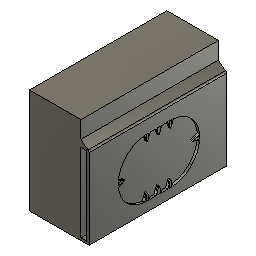
2nd mirror calibration holder with tabs (Autodesk Fusion 360 design; units mm, degrees)
Autodesk Fusion 360 part; units mm, degrees
sketch "Sketch1" plane through (0, 0, 0) normal (1, 0, 0) x (0, 0, -1)
  line L0 (0, 0) -> (-57, 0)
  line L1 (-57, 0) -> (-57, 54)
  line L2 (-57, 54) -> (0, 54)
  line L3 (0, 54) -> (0, 0)
  dimension "d1" = 57
  dimension "d2" = 54
  constraint horizontal L0
  constraint vertical L1
  constraint horizontal L2
  constraint vertical L3
  constraint coincident L0.start L3.end
  measures "d1" distance of L0.start L0.end
  measures "d2" distance of L0.start L2.end
extrude "Extrude1" add sketch "Sketch1" along normal blind 9 makes body 1
sketch "Sketch2" plane through (9, 0, 0) normal (1, 0, 0) x (0, 0, -1)
  line L0 (0, 54) -> (-57, 54)
  line L1 (-57, 54) -> (-57, 0)
  line L2 (-57, 0) -> (0, 0)
  line L3 (0, 0) -> (0, 54)
  circle A0 centre (-28, 27) radius 18.5
  circle A1 centre (-28, 27) radius 12.5 construction
  line L4 (-28, 27) -> (-23, 27) construction
  line L5 (-28, 27) -> (-33, 27) construction
  circle A2 centre (-23, 27) radius 12.5
  circle A3 centre (-33, 27) radius 12.5
  line L6 (-45.5, 27) -> (-42.5, 27)
  line L7 (-42.5, 27) -> (-45.4405, 28.218)
  line L8 (-42.5, 27) -> (-45.4405, 25.782)
  line L9 (-33, 17.5) -> (-31.782, 14.5595)
  line L10 (-33, 14.5) -> (-33, 17.5) construction
  line L11 (-33, 17.5) -> (-34.218, 14.5595)
  line L12 (-33, 39.5) -> (-33, 36.5) construction
  line L13 (-33, 36.5) -> (-34.218, 39.4405)
  line L14 (-33, 36.5) -> (-31.782, 39.4405)
  line L15 (-28, 36.5) -> (-29.218, 39.4405)
  line L16 (-28, 39.5) -> (-28, 36.5) construction
  line L17 (-28, 36.5) -> (-26.782, 39.4405)
  line L18 (-28, 17.5) -> (-29.218, 14.5595)
  line L19 (-28, 14.5) -> (-28, 17.5) construction
  line L20 (-28, 17.5) -> (-26.782, 14.5595)
  line L21 (-23, 36.5) -> (-24.218, 39.4405)
  line L22 (-23, 39.5) -> (-23, 36.5) construction
  line L23 (-23, 36.5) -> (-21.782, 39.4405)
  line L24 (-23, 17.5) -> (-24.218, 14.5595)
  line L25 (-23, 14.5) -> (-23, 17.5) construction
  line L26 (-23, 17.5) -> (-21.782, 14.5595)
  line L27 (-45.5, 27) -> (-42.5, 27) construction
  line L28 (-42.5, 27) -> (-45.4405, 28.218)
  line L29 (-42.5, 27) -> (-45.4405, 25.782)
  line L30 (-10.5, 27) -> (-13.5, 27) construction
  line L31 (-13.5, 27) -> (-10.5595, 25.782)
  line L32 (-13.5, 27) -> (-10.5595, 28.218)
  line L33 (-33, 39.5) -> (-23, 39.5)
  line L34 (-33, 14.5) -> (-23, 14.5)
  line L35 (-31.782, 14.5595) -> (-31.7574, 14.5)
  line L36 (-29.218, 14.5595) -> (-29.2426, 14.5)
  line L37 (-26.782, 14.5595) -> (-26.7574, 14.5)
  line L38 (-24.218, 14.5595) -> (-24.2426, 14.5)
  line L39 (-31.782, 39.4405) -> (-31.7574, 39.5)
  line L40 (-29.218, 39.4405) -> (-29.2426, 39.5)
  line L41 (-26.782, 39.4405) -> (-26.7574, 39.5)
  line L42 (-24.218, 39.4405) -> (-24.2426, 39.5)
  dimension "d5" = 37
  dimension "d6" = 25
  dimension "d127" = 5
  dimension "d128" = 5
  dimension "d129" = 25
  dimension "d130" = 25
  dimension "d131" = 45
  dimension "d132" = 3
  dimension "d133" = 45
  dimension "d134" = 3
  dimension "d135" = 45
  dimension "d136" = 3
  dimension "d140" = 45
  dimension "d141" = 3
  dimension "d142" = 45
  dimension "d143" = 3
  dimension "d144" = 45
  dimension "d145" = 3
  dimension "d146" = 45
  dimension "d147" = 3
  dimension "d148" = 45
  dimension "d149" = 3
  dimension "d150" = 3
  dimension "d151" = 45
  constraint concentric A0 A1
  constraint coincident A0.centre A1.centre
  constraint horizontal L4
  constraint parallel L4 L5
  constraint coincident L4.end A2.centre
  constraint coincident L5.end A3.centre
  constraint coincident A3 L6.start
  constraint horizontal L6
  constraint coincident A3 L7.end
  constraint collinear L5 L6
  constraint symmetric L7.start L6 L8.start
  constraint symmetric L9.start L11.start L10
  constraint symmetric L9.end L11.end L10
  constraint symmetric L13.start L14.start L12
  constraint symmetric L13.end L14.end L12
  constraint coincident A3 L12.start
  constraint coincident A3 L13.end
  constraint vertical L12
  constraint coincident A3 L14.end
  constraint coincident A3 L11.end
  constraint coincident A3 L10.start
  constraint coincident A3 L9.end
  constraint vertical L10
  constraint coincident A3 L8.end
  constraint equal L7 L8
  constraint symmetric L18.start L20.start L19
  constraint symmetric L18.end L20.end L19
  constraint symmetric L15.start L17.start L16
  constraint symmetric L15.end L17.end L16
  constraint vertical L16
  constraint vertical L19
  constraint symmetric L24.start L26.start L25
  constraint symmetric L24.end L26.end L25
  constraint symmetric L21.start L23.start L22
  constraint symmetric L21.end L23.end L22
  constraint vertical L22
  constraint vertical L25
  constraint horizontal L27
  constraint symmetric L6.end L7.start L27
  constraint equal L28 L29
  constraint coincident A1 L15.end
  constraint coincident A1 L16.start
  constraint coincident A1 L17.end
  constraint coincident A2 L21.end
  constraint coincident A2 L22.start
  constraint coincident A2 L23.end
  constraint coincident A2 L32.end
  constraint coincident A2 L30.start
  constraint coincident A2 L31.end
  constraint horizontal L30
  constraint symmetric L30 L31 L32
  constraint coincident L30.end L32
  constraint coincident L31.start L30
  constraint equal L31 L32
  constraint coincident A1 L18.end
  constraint coincident A1 L19.start
  constraint coincident A1 L20.end
  constraint coincident A2 L24.end
  constraint coincident A2 L25.start
  constraint coincident A2 L26.end
  constraint coincident L34 L35.end
  constraint parallel L9 L35
  constraint coincident L34 L36.end
  constraint parallel L18 L36
  constraint coincident L34 L37.end
  constraint parallel L20 L37
  constraint coincident L34 L38.end
  constraint parallel L24 L38
  constraint coincident L33 L39.end
  constraint parallel L14 L39
  constraint coincident L33 L40.end
  constraint parallel L15 L40
  constraint coincident L33 L41.end
  constraint parallel L17 L41
  constraint coincident L33 L42.end
  constraint parallel L21 L42
  measures "d5" diameter of A0
  measures "d6" diameter of A1
  measures "d127" distance of A0.centre L5.end
  measures "d128" distance of A0.centre L4.end
  measures "d129" diameter of A2
  measures "d130" diameter of A3
  measures "d131" angle of L7 L8
  measures "d132" distance of L6.start L6.end
  measures "d133" angle of L9 L11
  measures "d134" distance of L9.start L10.start
  measures "d135" angle of L13 L14
  measures "d136" distance of L12.end L12.start
  measures "d140" angle of L18 L20
  measures "d141" distance of L18.start L19.start
  measures "d142" angle of L15 L17
  measures "d143" distance of L16.start L15.start
  measures "d144" angle of L24 L26
  measures "d145" distance of L24.start L25.start
  measures "d146" angle of L21 L23
  measures "d147" distance of L21.start L22.start
  measures "d148" angle of L28 L29
  measures "d149" distance of L6.end L6.start
  measures "d150" distance of L30.end L30.start
  measures "d151" angle of L31 L32
extrude "Extrude16" cut sketch "Sketch2" against normal blind 1 contours A2 A3 L17 L20 L21 L23 L24 L26 L31 L32 | A2 L17 L33 L41 L42 | A2 L20 L34 L37 L38 | A2 A3 L15 L17 L18 L20 | A3 L15 L33 L39 L40 | A3 L18 L34 L35 L36 | A2 A3 L7 L8 L9 L11 L13 L14 L15 L18 L28 L29 bodies 1
sketch "Sketch3" plane through (9, 27, 28) normal (1, 0, 0) x (0, 0, -1)
  line L0 (-29.01, 27.5) -> (28.01, 27.5)
  line L1 (28.01, 27.5) -> (28.01, -26.5)
  line L2 (-29.01, 27.5) -> (-29.01, -26.5)
  line L3 (28, 27) -> (-29, 27)
  line L4 (-29, 27) -> (-29, -27)
  line L5 (28, -27) -> (28, 27)
  line L6 (-30.01, 28.5) -> (-30.01, -26.5)
  line L7 (-30.01, 28.5) -> (29.01, 28.5)
  line L8 (29.01, 28.5) -> (29.01, -26.5)
  line L9 (-30.01, -26.5) -> (-29.01, -26.5)
  line L10 (29.01, -26.5) -> (28.01, -26.5)
  dimension "d7" = 0.5
  dimension "d8" = 0.01
  dimension "d9" = 0.01
  dimension "d10" = 54
  dimension "d11" = -1
  constraint horizontal L0
  constraint perpendicular L0 L1
  constraint perpendicular L0 L2
  constraint equal L1 L2
  constraint perpendicular L2 L9
  constraint perpendicular L1 L10
  measures "d7" distance of L0 L3
  measures "d8" distance of L2 L4
  measures "d9" distance of L1 L5
  measures "d10" distance of L0.start L2.end
extrude "Extrude2" add sketch "Sketch3" along normal blind -9.8 and the other way blind -0.8 separate body makes body 2
sketch "Sketch4" plane through (0, 0, -0.01) normal (0, 0, 1) x (1, 0, 0)
  line L0 (9.8, 54.5) -> (-0.8, 54.5)
  line L1 (-0.8, 54.5) -> (-0.8, 0.5)
  line L2 (-0.8, 0.5) -> (9.8, 0.5)
  line L3 (9.8, 0.5) -> (9.8, 54.5)
  line L4 (0, 54.5) -> (0, 0.5)
  line L5 (9, 0.5) -> (9, 54.5)
extrude "Extrude3" add sketch "Sketch4" along normal blind 2 contours L0 L2 L3 L5 | L0 L1 L2 L4 bodies 2
sketch "Sketch5" plane through (0, 54.5, 0) normal (0, -1, 0) x (1, 0, 0)
  line L0 (9, 1.99) -> (9.8, 1.99)
  line L1 (0, 1.99) -> (0, -0.01)
  line L2 (0, -0.01) -> (9, -0.01)
  line L3 (9.8, 1.99) -> (9.8, 57.01)
  line L4 (9.8, 57.01) -> (-0.8, 57.01)
  line L5 (-0.8, 57.01) -> (-0.8, 1.99)
  line L6 (0, 57.01) -> (0, 1.99)
  line L7 (9, -0.01) -> (9, 1.99)
  line L8 (9, 1.99) -> (9, 57.01)
  line L9 (-0.8, 1.99) -> (0, 1.99)
extrude "Extrude4" add sketch "Sketch5" along normal blind 2 contours L4 L5 L6 L9 bodies 2
sketch "Sketch6" plane through (0, 0, 57.01) normal (0, 0, -1) x (-1, 0, 0)
  line L0 (0.8, 52.5) -> (0, 52.5)
  line L1 (0, 52.5) -> (0, 54.5)
  line L2 (0, 54.5) -> (-9.8, 54.5)
  line L3 (-9.8, 54.5) -> (-9.8, 0.5)
  line L4 (-9.8, 0.5) -> (0.8, 0.5)
  line L5 (0.8, 0.5) -> (0.8, 52.5)
  line L6 (0, 0.5) -> (0, 52.5)
  line L7 (-9, 54.5) -> (-9, 0.5)
extrude "Extrude5" add sketch "Sketch6" along normal blind 2 contours L0 L4 L5 L6 | L2 L3 L4 L7 bodies 2
sketch "Sketch16" plane through (0, 55.5, 0) normal (0, 1, 0) x (-1, 0, 0)
  line L0 (-9.8, -1.01) -> (0.8, -1.01)
  line L1 (0.8, -1.01) -> (0.8, 58.01)
  line L2 (0.8, 58.01) -> (-9.8, 58.01)
  line L3 (-9.8, 58.01) -> (-9.8, -1.01)
  line L4 (-9.8, 58.01) -> (-24.8, 58.01)
  line L5 (-24.8, 58.01) -> (-24.8, -1.01)
  line L6 (-24.8, -1.01) -> (-9.8, -1.01)
  line L7 (-9.8, -1.01) -> (-9.8, 58.01)
  dimension "d81" = 15
  constraint horizontal L4
  constraint vertical L5
  constraint horizontal L6
  constraint vertical L7
  constraint coincident L2.end L3.start
  constraint coincident L0.start L3.end
  measures "d81" distance of L2.end L4.end
extrude "Extrude18" add sketch "Sketch16" against normal blind 1 contours L3 L4 L5 L6 L7 bodies 2
sketch "Sketch17" plane through (0, 54.5, 0) normal (0, -1, 0) x (1, 0, 0)
  line L0 (9.8, 55.01) -> (9, 55.01)
  line L1 (9, 55.01) -> (9, 57.01)
  line L2 (9, 57.01) -> (0, 57.01)
  line L3 (0, 57.01) -> (0, -0.01)
  line L4 (0, -0.01) -> (9, -0.01)
  line L5 (9, -0.01) -> (9, 1.99)
  line L6 (9, 1.99) -> (9.8, 1.99)
  line L7 (9.8, 1.99) -> (9.8, -1.01)
  line L8 (9.8, -1.01) -> (24.8, -1.01)
  line L9 (24.8, -1.01) -> (24.8, 58.01)
  line L10 (24.8, 58.01) -> (9.8, 58.01)
  line L11 (9.8, 58.01) -> (9.8, 55.01)
  line L12 (24.8, -1.01) -> (9.8, -1.01)
  line L13 (9.8, -1.01) -> (9.8, -0.01)
  line L14 (9.8, -0.01) -> (24.8, -0.01)
  line L15 (24.8, -0.01) -> (24.8, -1.01)
  line L16 (24.8, 58.01) -> (9.8, 58.01)
  line L17 (9.8, 58.01) -> (9.8, 57.01)
  line L18 (9.8, 57.01) -> (24.8, 57.01)
  line L19 (24.8, 57.01) -> (24.8, 58.01)
  dimension "d84" = 1
  dimension "d85" = 1
  constraint horizontal L12
  constraint vertical L13
  constraint horizontal L14
  constraint vertical L15
  constraint coincident L7 L13.end
  constraint coincident L8.end L9.start
  constraint horizontal L16
  constraint vertical L17
  constraint horizontal L18
  constraint vertical L19
  constraint coincident L11 L17.end
  constraint coincident L9.end L10.start
  measures "d84" distance of L12 L14
  measures "d85" distance of L9.end L18.end
extrude "Extrude19" add sketch "Sketch17" along normal up to surface (54 mm away) contours L9 L10 L11 L16 L17 L18 L19 | L7 L8 L9 L12 L13 L14 L15 bodies 2
sketch "Sketch19" plane through (0, 54.5, 0) normal (0, -1, 0) x (1, 0, 0)
  line L0 (24.8, -0.01) -> (23.8, -0.01)
  line L1 (23.8, -0.01) -> (23.8, 57.01)
  line L2 (23.8, 57.01) -> (24.8, 57.01)
  line L3 (24.8, 57.01) -> (24.8, -0.01)
  line L4 (21.3, 57.7) -> (19.3, 57.7)
  line L5 (19.3, 57.7) -> (19.3, -0.01)
  line L6 (19.3, -0.01) -> (21.3, -0.01)
  line L7 (21.3, -0.01) -> (21.3, 57.7)
  line L8 (24.8, 57.01) -> (9.8, 57.01)
  line L9 (9.8, 57.01) -> (9.8, 55.01)
  line L10 (9.8, 55.01) -> (9, 55.01)
  line L11 (9, 55.01) -> (9, 57.01)
  line L12 (9, 57.01) -> (0, 57.01)
  line L13 (0, 57.01) -> (0, -0.01)
  line L14 (0, -0.01) -> (9, -0.01)
  line L15 (9, -0.01) -> (9, 1.99)
  line L16 (9, 1.99) -> (9.8, 1.99)
  line L17 (9.8, 1.99) -> (9.8, -0.01)
  line L18 (9.8, -0.01) -> (24.8, -0.01)
  line L19 (24.8, -0.01) -> (24.8, 57.01)
  dimension "d89" = 1
  dimension "d90" = 2
  dimension "d91" = 2.5
  constraint horizontal L0
  constraint vertical L1
  constraint horizontal L2
  constraint vertical L3
  constraint horizontal L4
  constraint vertical L5
  constraint horizontal L6
  constraint vertical L7
  constraint collinear L2 L8
  constraint collinear L0 L18
  constraint collinear L6 L18
  constraint collinear L3 L19
  measures "d89" distance of L1 L3
  measures "d90" distance of L5 L7
  measures "d91" distance of L1 L7
extrude "Extrude20" add sketch "Sketch19" along normal blind 60 contours L0 L1 L2 L3 L8 L18 L19 | L5 L6 L7 L8 L18 bodies 2
extrude "Extrude21" cut 1 faces at (8, 27, 19.8333) along direction (1, 0, 0) up to surface (1 mm away) from surface at 15.8 on bodies 1 bodies 2
sketch "Sketch25" plane through (0, 0, -0.01) normal (0, 0, 1) x (1, 0, 0)
  line L0 (21.3, 0.5) -> (23.8, 0.5)
  line L1 (23.8, 54.5) -> (21.3, 54.5)
  line L2 (24.8, 55.5) -> (24.8, 45.5)
  line L3 (24.8, 45.5) -> (21.3, 45.5)
  line L4 (21.3, 54.5) -> (21.3, 45.5)
  line L5 (24.8, 45.5) -> (24.8, 55.5)
  line L6 (24.8, 55.5) -> (24.8, 0.5)
  line L7 (-0.8, 55.5) -> (24.8, 55.5)
  line L8 (21.3, 54.5) -> (21.3, 55.5)
  line L9 (24.8, 55.5) -> (21.3, 55.5)
  line L10 (24.8, 10.5) -> (19.3, 10.5)
  line L11 (19.3, -5.5) -> (24.8, -5.5)
  line L12 (24.8, -5.5) -> (24.8, 10.5)
  line L13 (9.8, 0.5) -> (19.3, -5.5)
  line L14 (19.3, 0.5) -> (19.3, 54.5)
  line L15 (-0.8, 0.5) -> (24.8, 0.5)
  line L16 (9.8, 0.5) -> (9.8, 54.5)
  line L17 (19.3, 10.5) -> (9.8, 10.5)
  line L18 (9.8, 10.5) -> (9.8, 0.5)
  line L19 (9.8, 0.5) -> (19.3, 0.5)
  line L20 (19.3, 0.5) -> (19.3, 10.5)
  line L21 (9.8, 0.5) -> (9.8, 10.5)
  line L22 (23.8, 0.5) -> (23.8, 54.5)
  line L23 (21.3, 54.5) -> (21.3, 0.5)
  point P0 (19.3, -5.5)
  dimension "d119" = 10
  dimension "d120" = 10
  constraint coincident L1.end L4.start
  constraint coincident L2.end L6
  constraint coincident L2.start L7
  constraint coincident L7 L8.end
  constraint perpendicular L7 L8
  constraint perpendicular L5 L9
  constraint horizontal L3
  constraint horizontal L10
  constraint horizontal L11
  constraint vertical L12
  constraint coincident L6 L10.start
  constraint coincident P0 L11.start
  constraint coincident L10.end L14
  constraint coincident L13.start L15
  constraint coincident L13.start L16
  constraint horizontal L17
  constraint vertical L18
  constraint horizontal L19
  constraint vertical L20
  constraint coincident L13.start L16.start
  measures "d119" distance of L3 L7
  measures "d120" distance of L10 L15
extrude "Extrude26" cut sketch "Sketch25" along normal blind 65 and the other way blind 10 contours L0 L10 L15 L22 L23 | L0 L11 L12 L13 L15 L19 | L10 L14 L15 L20 L23 | L6 L10 L12 L15 L22 | L14 L15 L16 L17 L18 L19 L20 L21 | L1 L3 L4 L22 L23 | L1 L2 L3 L5 L6 L7 L8 L9 L22 bodies 2
sketch "Sketch26" plane through (0, 0, 58.01) normal (0, 0, 1) x (1, 0, 0)
  line L0 (21.3, 55.5) -> (-0.8, 55.5)
  line L1 (-0.8, 55.5) -> (-0.8, 0.5)
  line L2 (-0.8, 0.5) -> (9.8, 0.5)
  line L3 (24.8, 45.5) -> (21.3, 45.5)
  arc A0 (21.3, 48.178) -> (24.8, 45.5) centre (41.2309, 70.6003) ccw
  line L4 (24.8, 10.5) -> (19.3, 10.5)
  line L5 (19.3, 11.5) -> (24.8, 11.5)
  line L6 (24.8, 11.5) -> (24.8, 10.5)
  line L7 (9.8, 0.5) -> (9.8, 10.5)
  line L8 (19.3, 10.5) -> (19.3, 11.5)
  line L9 (24.8, 45.5) -> (21.3, 45.5)
  line L10 (21.3, 45.5) -> (21.3, 55.5)
  line L11 (9.8, 10.5) -> (24.8, 10.5)
  line L12 (24.8, 10.5) -> (24.8, 45.5)
  dimension "d116" = 30
  dimension "d124" = 5.5
  dimension "d125" = 1
  constraint perpendicular L4 L6
  constraint perpendicular L5 L8
  measures "d116" radius of A0
  measures "d124" distance of L6 L8
  measures "d125" distance of L4 L5
extrude "Extrude27" add sketch "Sketch26" against normal up to surface (59.02 mm away) contours L3 A0 L9 L10 | L4 L5 L6 L8 L11 L12 bodies 2
sketch "Sketch27" plane through (0, 0, 58.01) normal (0, 0, 1) x (1, 0, 0)
  line L0 (21.3, 48.178) -> (21.3, 55.5)
  line L1 (24.8, 10.5) -> (24.8, 45.5)
  line L2 (23.7987, 11.5) -> (21.2974, 11.5)
  line L3 (21.2974, 11.5) -> (21.2974, 45.1898)
  line L4 (21.2974, 45.1898) -> (23.7987, 45.1898)
  line L5 (23.7987, 45.1898) -> (23.7987, 11.5)
  line L6 (9.8, 10.5) -> (24.8, 10.5)
  line L7 (9.8, 10.5) -> (-0.8, 10.5)
  line L8 (-0.8, 10.5) -> (-0.8, 0.5)
  line L9 (-0.8, 0.5) -> (9.8, 0.5)
  line L10 (9.8, 0.5) -> (9.8, 10.5)
  arc A0 (21.3, 48.178) -> (24.8, 45.5) centre (41.2309, 70.6003) ccw
  line L11 (21.3, 55.5) -> (-0.8, 55.5)
  line L12 (-0.8, 55.5) -> (-0.8, 0.5)
  line L13 (-0.8, 0.5) -> (9.8, 0.5)
  line L14 (9.8, 0.5) -> (9.8, 10.5)
  dimension "d126" = 1
  constraint horizontal L2
  constraint vertical L3
  constraint horizontal L4
  constraint vertical L5
  constraint horizontal L7
  constraint vertical L8
  constraint horizontal L9
  constraint vertical L10
  constraint coincident L6.start L7.start
  measures "d126" distance of L2 L6
extrude "Extrude28" cut sketch "Sketch27" against normal blind 70 contours L7 L8 L9 L10 L12 L13 L14 | L2 L3 L4 L5 bodies 2
fillet "Fillet3" radius 1 1 edges at (24.8, 45.5, 28.5) on bodies 2
sketch "Sketch28" plane through (24.8, 0, 0) normal (1, 0, 0) x (0, 0, -1)
  line L0 (1.01, 44.9651) -> (-58.01, 44.9651)
  line L1 (-58.01, 44.9651) -> (-58.01, 10.5)
  line L2 (-58.01, 10.5) -> (1.01, 10.5)
  line L3 (1.01, 10.5) -> (1.01, 44.9651)
  arc A0 (-45.4405, 25.782) -> (-34.218, 14.5595) centre (-33, 27) ccw
  line L4 (-45.4405, 25.782) -> (-42.5, 27)
  line L5 (-42.5, 27) -> (-45.4405, 28.218)
  arc A1 (-34.218, 39.4405) -> (-45.4405, 28.218) centre (-33, 27) ccw
  line L6 (-34.218, 39.4405) -> (-33, 36.5)
  line L7 (-33, 36.5) -> (-31.7574, 39.5)
  line L8 (-31.7574, 39.5) -> (-29.2426, 39.5)
  line L9 (-29.2426, 39.5) -> (-28, 36.5)
  line L10 (-28, 36.5) -> (-26.7574, 39.5)
  line L11 (-26.7574, 39.5) -> (-24.2426, 39.5)
  line L12 (-24.2426, 39.5) -> (-23, 36.5)
  line L13 (-23, 36.5) -> (-21.782, 39.4405)
  arc A2 (-10.5595, 28.218) -> (-21.782, 39.4405) centre (-23, 27) ccw
  line L14 (-10.5595, 28.218) -> (-13.5, 27)
  line L15 (-13.5, 27) -> (-10.5595, 25.782)
  arc A3 (-21.782, 14.5595) -> (-10.5595, 25.782) centre (-23, 27) ccw
  line L16 (-21.782, 14.5595) -> (-23, 17.5)
  line L17 (-23, 17.5) -> (-24.2426, 14.5)
  line L18 (-24.2426, 14.5) -> (-26.7574, 14.5)
  line L19 (-26.7574, 14.5) -> (-28, 17.5)
  line L20 (-28, 17.5) -> (-29.2426, 14.5)
  line L21 (-29.2426, 14.5) -> (-31.7574, 14.5)
  line L22 (-31.7574, 14.5) -> (-33, 17.5)
  line L23 (-33, 17.5) -> (-34.218, 14.5595)
  line L24 (-45.4405, 39.5) -> (-10.5595, 39.5)
  line L25 (-10.5595, 39.5) -> (-10.5595, 14.5)
  line L26 (-10.5595, 14.5) -> (-45.4405, 14.5)
  line L27 (-45.4405, 14.5) -> (-45.4405, 39.5)
  line L28 (-42.5, 27.5) -> (-45.4405, 27.5)
  line L29 (-45.4405, 27.5) -> (-45.4405, 26.5)
  line L30 (-45.4405, 26.5) -> (-42.5, 26.5)
  line L31 (-42.5, 26.5) -> (-42.5, 27.5)
  line L32 (-33.5, 17.5) -> (-33.5, 14.5)
  line L33 (-32.5, 17.5) -> (-33.5, 17.5)
  line L34 (-32.5, 14.5) -> (-32.5, 17.5)
  line L35 (-33.5, 39.5) -> (-33.5, 36.5)
  line L36 (-32.5, 36.5) -> (-32.5, 39.5)
  line L37 (-33.5, 36.5) -> (-32.5, 36.5)
  line L38 (-28.5, 17.5) -> (-28.5, 14.5)
  line L39 (-27.5, 14.5) -> (-27.5, 17.5)
  line L40 (-27.5, 17.5) -> (-28.5, 17.5)
  line L41 (-28.5, 39.5) -> (-28.5, 36.5)
  line L42 (-28.5, 36.5) -> (-27.5, 36.5)
  line L43 (-27.5, 36.5) -> (-27.5, 39.5)
  line L44 (-23.5, 17.5) -> (-23.5, 14.5)
  line L45 (-22.5, 17.5) -> (-23.5, 17.5)
  line L46 (-22.5, 14.5) -> (-22.5, 17.5)
  line L47 (-23.5, 39.5) -> (-23.5, 36.5)
  line L48 (-23.5, 36.5) -> (-22.5, 36.5)
  line L49 (-22.5, 36.5) -> (-22.5, 39.5)
  line L50 (-28, 17.5) -> (-28, 36.5) construction
  line L51 (-13.5, 26.5) -> (-13.5, 27.5)
  line L52 (-13.5, 27.5) -> (-10.5595, 27.5)
  line L53 (-10.5595, 26.5) -> (-13.5, 26.5)
  dimension "d153" = 1
  dimension "d154" = 1
  dimension "d155" = 1
  dimension "d156" = 1
  dimension "d157" = 1
  dimension "d158" = 1
  dimension "d159" = 1
  constraint horizontal L24
  constraint vertical L25
  constraint horizontal L26
  constraint vertical L27
  constraint collinear L21 L26
  constraint coincident L5.end L27
  constraint coincident A2.start L25
  constraint collinear L8 L24
  constraint horizontal L28
  constraint vertical L29
  constraint horizontal L30
  constraint vertical L31
  constraint coincident L27 L29.end
  constraint midpoint L4.end L31
  constraint coincident L19.end L20.start
  constraint coincident L9.end L10.start
  constraint symmetric L28.start L50 L51.end
  constraint symmetric L28.end L50 L52.end
  constraint symmetric L29.end L50 L53.start
  constraint symmetric L30.end L50 L51.start
  constraint midpoint L6.end L37
  constraint coincident L24 L36.end
  constraint coincident L24 L35.start
  constraint perpendicular L24 L35
  constraint perpendicular L24 L36
  constraint horizontal L37
  constraint horizontal L42
  constraint horizontal L48
  constraint vertical L41
  constraint vertical L43
  constraint vertical L47
  constraint vertical L49
  constraint vertical L32
  constraint vertical L34
  constraint horizontal L33
  constraint horizontal L40
  constraint vertical L39
  constraint vertical L38
  constraint vertical L44
  constraint vertical L46
  constraint horizontal L45
  constraint midpoint L42 L9.end
  constraint midpoint L12.end L48
  constraint midpoint L16.end L45
  constraint midpoint L40 L19.end
  constraint midpoint L22.end L33
  constraint coincident L26 L34.start
  constraint coincident L26 L32.end
  constraint coincident L26 L38.end
  constraint coincident L26 L39.start
  constraint coincident L26 L44.end
  constraint coincident L26 L46.start
  constraint coincident L24 L41.start
  constraint coincident L24 L43.end
  constraint coincident L24 L47.start
  constraint coincident L24 L49.end
  measures "d153" distance of L28.start L30.end
  measures "d154" distance of L33.start L32.start
  measures "d155" distance of L35.end L36.start
  measures "d156" distance of L39.end L38.start
  measures "d157" distance of L42.end L41.end
  measures "d158" distance of L44.start L45.start
  measures "d159" distance of L48.end L47.end
extrude "Extrude29" cut sketch "Sketch28" against normal blind 0.5 contours L4 L5 L27 L28 L29 L30 | L22 L23 L26 L32 L34 | L6 L7 L24 L35 L36 | L19 L20 L26 L38 L39 | L9 L10 L24 L41 L43 | L16 L17 L26 L44 L46 | L12 L13 L24 L47 L49 | L14 L15 L25 L52 L53 bodies 2
extrude "Extrude30" add sketch "Sketch28" against normal blind 0.5 separate body contours L4 L5 L27 L28 L29 L30 | L22 L23 L26 L32 L34 | L6 L7 L24 L35 L36 | L19 L20 L26 L38 L39 | L9 L10 L24 L41 L43 | L16 L17 L26 L44 L46 | L12 L13 L24 L47 L49 | L14 L15 L25 L52 L53 makes body 3 at (24.8, 15.6953, 23.1667) makes body 4 at (24.8, 38.3047, 33.1667) makes body 5 at (24.8, 38.3047, 28.1667) makes body 6 at (24.8, 15.6953, 28.1667) makes body 7 at (24.8, 27.1667, 11.7151) makes body 8 at (24.8, 26.8333, 44.2849) makes body 9 at (24.8, 38.3047, 23.1667) makes body 10 at (24.8, 15.6953, 33.1667)
copy_body "Body->Comp1" bodies 2 removing the originals makes body 11 in component "Alignment tool"
copy_body "Body->Comp2" bodies 3 removing the originals makes body 12 in component "Inlays"
copy_body "CutPasteBodies1" bodies 4 5 6 7 8 9 10 removing the originals makes body 13 makes body 14 makes body 15 makes body 16 makes body 17 makes body 18 makes body 19 in component "Inlays"
copy_body "CutPasteBodies2" bodies 11 removing the originals makes body 20 in component "Inlays"
component "Alignment tool" placed x (1, 0, 0) y (0, 1, 0) z (0, 0, 1) at (0, 0, 0)
component "Inlays" placed x (1, 0, 0) y (0, 1, 0) z (0, 0, 1) at (0, 0, 0)
hidden bodies 1
equation "d9 = d8"
equation "d12 = -9 mm - edge_thickness"
equation "d14 = -edge_thickness"
equation "d16 = -edge_thickness"
equation "d17 = edge_stickout"
equation "d19 = -edge_thickness"
equation "d20 = edge_stickout"
equation "d22 = -edge_thickness"
equation "edge_thickness = 0.8 mm"
equation "edge_stickout = 2 mm"
equation "d25 = edge_stickout"
equation "d27 = -edge_thickness"
equation "d28 = -edge_thickness"
equation "d29 = -edge_thickness"
equation "slit = 2 mm"
equation "d85 = d84"
equation "d120 = d119"
equation "d127 = tab_spacing"
equation "d128 = tab_spacing"
equation "d131 = tab_angle"
equation "d132 = tab_length"
equation "d133 = tab_angle"
equation "d134 = tab_length"
equation "d135 = tab_angle"
equation "d136 = tab_length"
equation "tab_length = 3 mm"
equation "tab_spacing = 5 mm"
equation "tab_angle = 45 deg"
equation "d140 = tab_angle"
equation "d141 = tab_length"
equation "d142 = tab_angle"
equation "d143 = tab_length"
equation "d144 = tab_angle"
equation "d145 = tab_length"
equation "d146 = tab_angle"
equation "d147 = tab_length"
equation "d148 = tab_angle"
equation "d149 = tab_length"
equation "d150 = tab_length"
equation "d151 = tab_angle"
equation "tab_inlay_width = 1 mm"
equation "d153 = tab_inlay_width"
equation "d154 = tab_inlay_width"
equation "d155 = tab_inlay_width"
equation "d156 = tab_inlay_width"
equation "d157 = tab_inlay_width"
equation "d158 = tab_inlay_width"
equation "d159 = tab_inlay_width"
